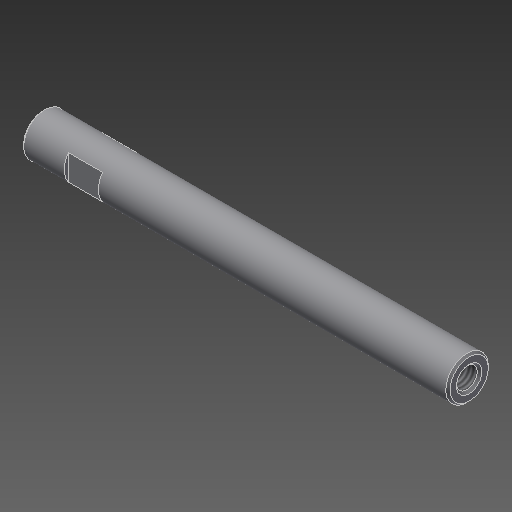
# Autodesk Inventor part: PSPWR10-100-M5-N6-SC10
Saved by Autodesk Inventor 2021.1 (Build 251245010, 245A)
## iProperties
Created: 2010-03-11
Part Number: PSPWR10-100-M5-N6-SC10
Catalog Web Link: www.cadenas.de
Document SubType Name: Modeling
Density: 1 g/cm^3
Material: MISUMI
Appearance: 既定
Category: PARTsolutions
NB: PSPWR10-100-M5-N6-SC10
NN: SPWR, SSPWR, RSPWR, PSPWR
NT: Precision Linear Shafts - Both Ends Female Thread Pipe Wrench Flat Type
NBSYN: $PN.
LINA: PSPWR10-100-M5-N6-SC10
PN: PSPWR10-100-M5-N6-SC10
TYPE: PSPWR
MAT: 0
MATALG: '0','SUJ2(52100 Bearing Steel)(1.3505_100Cr6)', '1','SUS440C(440C Stainless Steel)(1.4125_X105CrMo17)'
HT: Induction Hardening 58 HRC~
ST: 1
STALG: '0','-', '2' , 'Low Temperature Black Chrome Plating' , '1','Hard Chrome Plating >=5µ'
D: 10
ALT1ALG: '', 'w/o DKC (Outer Dia. Tolerance (High Precision Class))', '-DKC','with DKC (Outer Dia. Tolerance (High Precision Class))'
DTOL: -0.005/-0.014
M: 5
MALG: '5','5','6','6'
MMD: 5.000
MMIN: 4.134
N: 6
NALG: '5','5','6','6'
NMD: 6.000
NMIN: 4.917
L: 100.0
LMAX: 800.0
LMAX1: 800.0
LMAX2: 400.0
LMIN: 30.000
LMIN1: 30.000
LMIN2: 20.0
LTOL: 0
INCR: 1.0
C1: 0.5
SC: 10
SC1: [10:80/1]
SC2: 92
SC3: 10
SC4: 80
SC5: 92.000
W: 8
LL1: 8
DP: 9
PITCH: 1.000
L3: 100.000
L4: 0.000
LT: 100.0
LLM: 0.000
LLN: 0.000
LM: 10.000
LN: 12.000
LMIN3: 88.000
DD: 4
C: 0.5 or Less
THREAD: 1
MMD1: 10.000
NMD1: 12.000
TH: 0
TH1: 0
KT: DUMMY
PSOL_IDENT_0: {\\partserver002.servicenet\dplatte\cadenas\23d-libs\misumi_usa_inc\metric\precision_linear_shafts\s
PSOL_IDENT_1: pwr.prj},231 {VTYP=3D},{NB=PSPWR10-100-M5-N6-SC10},{LINA=PSPWR10-100-M5-N6-SC10},{NN=SPWR, SSPWR, RS
PSOL_IDENT_2: PWR, PSPWR},{DATE=13.10.2009 15:32:20},{GEOMDATE=17.08.2009 00:00:00},{VERSION=},{LINEID=110},{LINES
PSOL_IDENT_3: UBID=-1},{WBVAR=MAT,ST,ALT1,M,N,ALT2,L,SC}  {NB=PSPWR10-100-M5-N6-SC10},{LINA=PSPWR10-100-M5-N6-SC10
PSOL_IDENT_4: },{KT=DUMMY},{PN=PSPWR10-100-M5-N6-SC10},{TYPE=PSPWR},{MAT=0},{MATALG='0','SUJ2(52100 Bearing Steel)
PSOL_IDENT_5: (1.3505_100Cr6)', '1','SUS440C(440C Stainless Steel)(1.4125_X105CrMo17)'},{HT=Induction Hardening 58
PSOL_IDENT_6: HRC~},{ST=1},{STALG= '0','-', '2' , 'Low Temperature Black Chrome Plating' , '1','Hard Chrome Plati
PSOL_IDENT_7: ng >=5µ' },{D=10},{ALT1=},{ALT1ALG='', 'w/o DKC (Outer Dia. Tolerance (High Precision Class))', '-DK
PSOL_IDENT_8: C','with DKC (Outer Dia. Tolerance (High Precision Class))'},{DTOL=-0.005/-0.014},{M=5},{MALG='5','5
PSOL_IDENT_9: ','6','6'},{MMD=5},{MMIN=4.134},{N=6},{NALG='5','5','6','6'},{NMD=6},{NMIN=4.917},{ALT2=},{L=100.0},
PSOL_IDENT_10: {LMAX=800.0},{LMAX1=800.0},{LMAX2=400.0},{LMIN=30},{LMIN1=30},{LMIN2=20.0},{LTOL=0},{INCR=1.0},{C1=0
PSOL_IDENT_11: .5},{SC=10},{SC1=[10:80/1]},{SC2=92},{SC3=10},{SC4=80},{SC5=92},{W=8},{LL1=8},{DP=9},{PITCH=1},{L3=1
PSOL_IDENT_12: 00},{L4=0},{LT=100.0},{LLM=0},{LLN=0},{LM=10},{LN=12},{LMIN3=88},{DD=4},{C=0.5 or Less},{THREAD=1},{
PSOL_IDENT_13: MMD1=10},{NMD1=12},{TH=0},{TH1=0}
Title: シャフト
Comments: Precision Linear Shafts - Both Ends Female Thread Pipe Wrench Flat Type
Autodesk Inventor part; units mm, degrees
ref_plane "YZ Plane" through (0, 0, 0) normal (1, 0, 0) x (0, 1, 0)
ref_plane "XZ Plane" through (0, 0, 0) normal (0, 1, 0) x (-1, 0, 0)
ref_plane "XY Plane" through (0, 0, 0) normal (0, 0, 1) x (1, 0, 0)
sketch "Sketch_1" plane through (0, 0, 0) normal (0, 0, 1) x (1, 0, 0)
  line L0 (100, 0) -> (0, 0)
  line L1 (0, 4.5) -> (0, 2)
  line L2 (0, 2) -> (100, 2)
  line L3 (100, 2) -> (100, 4.5)
  line L4 (100, 4.5) -> (99.5, 5)
  line L5 (99.5, 5) -> (0.5, 5)
  line L6 (0.5, 5) -> (0, 4.5)
  constraints: 14 end point
revolve "Revolution1" add sketch "Sketch_1" angle 360 about axis through (100, 0, 0) along (1, 0, 0)
sketch "Sketch_6" plane through (0, 0, 0) normal (0, 0, 1) x (1, 0, 0)
  line L0 (12.5, 0) -> (0, 0)
  line L1 (0, 0) -> (0, 2.5)
  line L2 (0, 2.5) -> (0.433, 2.067)
  line L3 (0.433, 2.067) -> (11.3066, 2.067)
  line L4 (11.3066, 2.067) -> (12.5, 0)
  line L5 (12.5, 0) -> (0, 0)
  constraints: 12 end point
revolve "Revolution2" cut sketch "Sketch_6" angle 360 about axis through (12.5, 0, 0) along (1, 0, 0)
thread "Thread1" size "M5x0.8" class "6H" standard "ISO Metric profile" length 10 offset 1.3066
sketch "Sketch_7" plane through (0, 0, 0) normal (0, 0, 1) x (1, 0, 0)
  line L0 (100, 0) -> (85, 0)
  line L1 (85, 0) -> (86.4194, 2.4585)
  line L2 (86.4194, 2.4585) -> (99.4585, 2.4585)
  line L3 (99.4585, 2.4585) -> (100, 3)
  line L4 (100, 3) -> (100, 0)
  line L5 (100, 0) -> (85, 0)
  constraints: 12 end point
revolve "Revolution3" cut sketch "Sketch_7" angle 360 about axis through (100, 0, 0) along (1, 0, 0)
thread "Thread2" size "M6x1" class "6H" standard "ISO Metric profile" length 12 offset 1.5806
sketch "Sketch_2" plane through (10, 0, 0) normal (1, 0, 0) x (0, 0, -1)
  line L0 (-6, 7) -> (-6, -5)
  line L1 (-6, -5) -> (-4, -5)
  line L2 (-4, -5) -> (-4, 6)
  line L3 (-4, 6) -> (4, 6)
  line L4 (4, 6) -> (4, -5)
  line L5 (4, -5) -> (6, -5)
  line L6 (6, -5) -> (6, 7)
  line L7 (6, 7) -> (-6, 7)
  constraints: 16 end point
extrude "Extrusion1" cut sketch "Sketch_2" along normal blind 8
